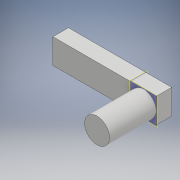
# Autodesk Inventor part: Palanca
Saved by Autodesk Inventor 2017 SP1 (Build 210196100, 196)
## iProperties
Part Number: Palanca
Material: Genérico
Document SubType Name: Modeling
Designer: Juan
Density: 1 g/cm^3
Appearance: Valor por defecto
Author: Juan
Autodesk Inventor part; units mm, degrees
ref_plane "YZ Plane" through (0, 0, 0) normal (1, 0, 0) x (0, 1, 0)
ref_plane "XZ Plane" through (0, 0, 0) normal (0, 1, 0) x (-1, 0, 0)
ref_plane "XY Plane" through (0, 0, 0) normal (0, 0, 1) x (1, 0, 0)
sketch "Boceto1" plane through (0, 0, 0) normal (0, 1, 0) x (-1, 0, 0)
  circle A0 centre (0, 0) radius 4
  dimension "d0" = 8
  constraints: 1 centre point, 1 coincident
  measures "d0" diameter of A0
extrude "Extrusión1" add sketch "Boceto1" along normal blind 15
ref_plane "Plano de trabajo1" through (0, 15, 0) normal (0, 1, 0) x (1, 0, 0)
sketch "Boceto2" plane through (0, 15, 0) normal (0, 1, 0) x (1, 0, 0)
  circle A0 centre (0, 0) radius 4 construction
  line L0 (0, -4) -> (-4.1758, -4) construction
  line L1 (-4.1758, -4) -> (-4.1758, 4) construction
  line L2 (-4.1758, 4) -> (4, 4) construction
  line L3 (4, 4) -> (4, -4) construction
  line L4 (4, -4) -> (0, -4) construction
  line L5 (-4.1758, -4) -> (-4.1758, 4)
  line L6 (4, 4) -> (4, -4)
  line L7 (-4.1758, -4) -> (4, -4)
  line L8 (-4.1758, 4) -> (4, 4)
  constraints: 18 end point, 5 perpendicular, 3 equal length, 3 horizontal, 1 point on line, 1 vertical alignment, 1 other
extrude "Extrusión2" add sketch "Boceto2" along normal blind 5
ref_plane "Plano de trabajo2" through (-4.1758, 15, -4) normal (-1, 0, 0) x (0, 0, 1)
sketch "Boceto3" plane through (-4.1758, 15, -4) normal (-1, 0, 0) x (0, 0, 1)
  line L0 (0, 5) -> (8, 5) projected
  line L1 (0, 5) -> (8, 5)
  line L2 (8, 0) -> (8, 5) projected
  line L3 (8, 5) -> (8, 0)
  line L4 (8, 0) -> (0, 0) projected
  line L5 (8, 0) -> (0, 0)
  line L6 (0, 0) -> (0, 5) projected
  line L7 (0, 0) -> (0, 5)
  point P0 (4, -15)
  constraints: 8 end point, 3 collinear, 1 perpendicular
extrude "Extrusión3" add sketch "Boceto3" along normal blind 25
